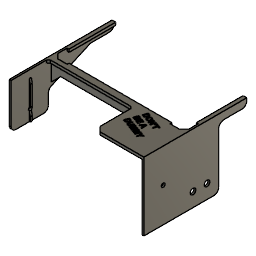
MEANWELL BRACKET (Autodesk Fusion 360 design; units mm, degrees)
Autodesk Fusion 360 part; units mm, degrees
sketch "Sketch1" plane through (0, 0, 0) normal (0, 0, 1) x (1, 0, 0)
  line L0 (95, 0) -> (140, 0)
  line L1 (140, 0) -> (140, 110)
  line L2 (0, 110) -> (0, 0)
  line L3 (90, 5) -> (90, 38)
  line L4 (88, 40) -> (2, 40)
  line L5 (0, 38) -> (0, 0)
  line L6 (0, 110) -> (-2, 110)
  line L7 (-2, 110) -> (-2, 0)
  line L8 (-2, 0) -> (0, 0)
  line L9 (0, 0) -> (0, 110)
  line L10 (140, 0) -> (142, 0)
  line L11 (142, 0) -> (142, 110)
  line L12 (142, 110) -> (140, 110)
  line L13 (140, 110) -> (140, 0)
  line L14 (140, 110) -> (140, 50)
  line L15 (135, 45) -> (5, 45)
  line L16 (0, 50) -> (0, 110)
  line L17 (140, 50) -> (135, 45)
  line L18 (5, 45) -> (0, 50)
  line L19 (90, 38) -> (88, 40)
  line L20 (2, 40) -> (0, 38)
  line L21 (90, 5) -> (95, 0)
  line L22 (0, 45) -> (140, 45)
  line L23 (140, 45) -> (140, 43)
  line L24 (140, 43) -> (0, 43)
  line L25 (0, 43) -> (0, 45)
  line L26 (0, 110) -> (2, 110)
  line L27 (2, 110) -> (2, 60)
  line L28 (2, 60) -> (0, 60)
  line L29 (0, 60) -> (0, 110)
  line L30 (140, 110) -> (138, 110)
  line L31 (138, 110) -> (138, 60)
  line L32 (138, 60) -> (140, 60)
  line L33 (140, 60) -> (140, 110)
  line L34 (5, 45) -> (15, 45)
  line L35 (135, 45) -> (125, 45)
  line L36 (15, 45) -> (125, 45)
  line L37 (125, 45) -> (125, 47)
  line L38 (125, 47) -> (15, 47)
  line L39 (15, 47) -> (15, 45)
  point P0 (90, 0)
  point P1 (90, 40)
  point P2 (0, 40)
  point P3 (140, 45)
  point P4 (0, 45)
  dimension "d1" = 140
  dimension "d2" = 110
  dimension "d3" = 90
  dimension "d4" = 40
  dimension "d5" = 2
  dimension "d6" = 110
  dimension "d7" = 2
  dimension "d8" = 110
  dimension "d9" = 65
  dimension "d10" = 5
  dimension "d11" = 5
  dimension "d12" = 5
  dimension "d13" = 5
  dimension "d14" = 2
  dimension "d15" = 2
  dimension "d16" = 2
  dimension "d17" = 2
  dimension "d18" = 5
  dimension "d19" = 5
  dimension "d22" = 2
  dimension "d23" = 50
  dimension "d24" = 2
  dimension "d25" = 50
  dimension "d26" = 10
  dimension "d27" = 10
  dimension "d28" = 110
  dimension "d29" = 2
  constraint horizontal L0
  constraint vertical L1
  constraint vertical L2
  constraint coincident L2.end L5.end
  constraint vertical L3
  constraint horizontal L4
  constraint vertical L5
  constraint horizontal L6
  constraint vertical L7
  constraint horizontal L8
  constraint vertical L9
  constraint horizontal L10
  constraint vertical L11
  constraint horizontal L12
  constraint vertical L13
  constraint vertical L14
  constraint horizontal L15
  constraint vertical L16
  constraint coincident L1 P3
  constraint coincident P3 L14
  constraint coincident P3 L15
  constraint coincident P4 L15
  constraint coincident P4 L16
  constraint coincident P1 L3
  constraint coincident P1 L4
  constraint coincident P2 L4
  constraint coincident P2 L5
  constraint coincident P0 L3
  constraint coincident L0 P0
  constraint horizontal L22
  constraint vertical L23
  constraint horizontal L24
  constraint vertical L25
  constraint coincident L13 L23.end
  constraint coincident P4 L22.start
  constraint horizontal L26
  constraint vertical L27
  constraint horizontal L28
  constraint vertical L29
  constraint horizontal L30
  constraint vertical L31
  constraint horizontal L32
  constraint vertical L33
  constraint parallel L22 L34
  constraint parallel L22 L35
  constraint horizontal L36
  constraint vertical L37
  constraint horizontal L38
  constraint vertical L39
  measures "d1" distance of L2.end L0.end
  measures "d2" distance of L2.end L2.start
  measures "d3" distance of L2.end P0
  measures "d4" distance of L2.end P2
  measures "d5" distance of L2.start L6.end
  measures "d6" distance of L2.start L2.end
  measures "d7" distance of L0.end L10.end
  measures "d8" distance of L0.end L1.end
  measures "d9" distance of L2.start L22.start
  measures "d10" distance of P3 L14.end
  measures "d11" distance of P3 L15.start
  measures "d12" distance of P4 L15.end
  measures "d13" distance of P4 L16.start
  measures "d14" distance of P1 L3.end
  measures "d15" distance of P1 L4.start
  measures "d16" distance of P2 L4.end
  measures "d17" distance of P2 L5.start
  measures "d18" distance of P0 L3.start
  measures "d19" distance of P0 L0.start
  measures "d22" distance of L2.start L26.end
  measures "d23" distance of L2.start L28.end
  measures "d24" distance of L1.end L30.end
  measures "d25" distance of L1.end L32.end
  measures "d26" distance of L15.end L34.end
  measures "d27" distance of L15.start L35.end
  measures "d28" distance of L34.end L35.end
  measures "d29" distance of L34.end L38.end
extrude "Extrude1" add sketch "Sketch1" along normal blind 3
extrude "Extrude2" add sketch "Sketch1" against normal blind 10 contours L1 L2 L9 L13 L15 L22 L23 L24 L25 L34 L35 L36
extrude "Extrude3" add sketch "Sketch1" against normal blind 45 contours L1 L10 L11 L12 L13 L14 L23 L33 | L2 L5 L6 L7 L8 L9 L16 L25 L29
sketch "Sketch2" plane through (0, 0, 0) normal (1, 0, 0) x (0, 1, 0)
  line L0 (110, -45) -> (40, -45)
  line L1 (40, -45) -> (40, -25)
  line L2 (85, -5) -> (110, -5)
  line L3 (110, -5) -> (110, -45)
  line L4 (40, -25) -> (85, -5)
  point P0 (40, -5)
  dimension "d34" = 70
  dimension "d35" = 40
  dimension "d36" = 20
  dimension "d37" = 45
  constraint horizontal L0
  constraint vertical L1
  constraint horizontal L2
  constraint vertical L3
  constraint coincident P0 L1
  constraint coincident P0 L2
  measures "d34" distance of L0.start L0.end
  measures "d35" distance of L0.start L2.end
  measures "d36" distance of P0 L1.end
  measures "d37" distance of P0 L2.start
extrude "Extrude4" cut sketch "Sketch2" along normal blind 210 and the other way blind 40
sketch "Sketch3" plane through (0, 0, 0) normal (1, 0, 0) x (0, 1, 0)
  line L0 (0, 0) -> (0, -15)
  line L1 (0, -33.26) -> (0, -15)
  circle A0 centre (20.65, -33.26) radius 2
  line L2 (21.65, -34.9921) -> (21.65, -45)
  line L3 (21.65, -45) -> (20.65, -45)
  line L4 (19.65, -34.9921) -> (19.65, -45)
  line L5 (19.65, -45) -> (20.65, -45)
  line L6 (19.65, -45) -> (21.65, -45)
  line L7 (21.65, -5) -> (19.65, -5)
  line L8 (19.65, -5) -> (19.65, -31.5279)
  line L9 (19.65, -34.9921) -> (19.65, -45)
  line L10 (21.65, -45) -> (21.65, -34.9921)
  line L11 (21.65, -31.5279) -> (21.65, -5)
  dimension "d42" = 15
  dimension "d44" = 18.26
  dimension "d45" = 4
  dimension "d54" = 2
  dimension "d55" = 40
  constraint coincident L0.start origin
  constraint vertical L0
  constraint vertical L1
  constraint vertical L2
  constraint horizontal L3
  constraint vertical L4
  constraint horizontal L5
  constraint horizontal L6
  constraint vertical L10
  constraint horizontal L7
  constraint vertical L8
  constraint coincident A0 L8.end
  constraint coincident A0 L4.start
  constraint collinear L8 L9
  constraint coincident A0 L2.start
  constraint coincident A0 L11.start
  constraint collinear L10 L11
  measures "d42" distance of L0.start L0.end
  measures "d44" distance of L0.end L1.start
  measures "d45" diameter of A0
  measures "d54" distance of L4.end L2.end
  measures "d55" distance of L4.end L7.end
extrude "Extrude5" cut sketch "Sketch3" along normal blind 175 and the other way blind 15 contours A0
fillet "Fillet1" radius 5 10 edges at (141, 40, -45) (141, 40, -25) (141, 85, -5) (141, 110, -5) (141, 0, -45) (-1, 0, -45) (-1, 40, -45) (-1, 40, -25) (-1, 85, -5) (-1, 110, -5)
extrude "Extrude6" add sketch "Sketch3" along normal blind 1 contours A0 L7 L8 L11 | A0 L2 L3 L4 L5 L6 L9 L10
chamfer "Chamfer1" distance 5 distance2 1 1 edges at (1, 20.65, -5) measured on face at (1, 20.6002, -13.7552)
chamfer "Chamfer2" distance 4.5 distance2 1 1 edges at (1, 20.65, -35.26) measured on face at (1, 20.6998, -41.7515)
ref_plane "WorkPlane1" through (70, 55, -21) normal (1, 0, 0) x (0, 1, 0)
mirror "Mirror1" about plane through (70, 55, -21) normal (1, 0, 0) of "Extrude6"
chamfer "Chamfer3" distance 1 distance2 5 1 edges at (139, 20.65, -5) measured on face at (139.6667, 20.9833, -5)
chamfer "Chamfer3" distance 1 distance2 5 1 edges at (139, 20.65, -35.26) measured on face at (140.3333, 19.8274, -31.437)
sketch "Sketch4" plane through (142, 0, 0) normal (1, 0, 0) x (0, 1, 0)
  circle A0 centre (20.65, -33.26) radius 2
  arc A1 (0, -40) -> (5, -45) centre (5, -40) ccw
  line L0 (5, -45) -> (35, -45)
  arc A2 (35, -45) -> (40, -40) centre (35, -40) ccw
  line L1 (40, -40) -> (40, -28.2494)
  arc A3 (42.9693, -23.6803) -> (40, -28.2494) centre (45, -28.2494) ccw
  line L2 (42.9693, -23.6803) -> (84.0304, -5.4309)
  arc A4 (86.0611, -5) -> (84.0304, -5.4309) centre (86.0611, -10) ccw
  line L3 (86.0611, -5) -> (105, -5)
  arc A5 (105, -5) -> (110, 0) centre (105, 0) ccw
  line L4 (110, 0) -> (110, 3)
  line L5 (110, 3) -> (0, 3)
  line L6 (0, 3) -> (0, -40)
  line L7 (0, -40) -> (35, -40)
  line L8 (80, -40) -> (80, -70)
  line L9 (80, -70) -> (0, -70)
  line L10 (0, -70) -> (0, -40)
  line L11 (35, -40) -> (35, -5)
  line L12 (35, -5) -> (80, -5)
  line L13 (80, -5) -> (80, -40)
  line L14 (0, -70) -> (67.5, -70)
  line L15 (67.5, -70) -> (67.5, -55)
  line L16 (67.5, -55) -> (0, -55)
  line L17 (0, -55) -> (0, -70)
  line L18 (67.5, -55) -> (52.5, -55)
  circle A6 centre (52.5, -55) radius 3
  circle A7 centre (67.5, -55) radius 3
  dimension "d68" = 80
  dimension "d69" = 30
  dimension "d70" = 45
  dimension "d71" = 35
  dimension "d76" = 67.5
  dimension "d77" = 15
  dimension "d78" = 15
  dimension "d79" = 6
  dimension "d80" = 6
  constraint horizontal L7
  constraint vertical L8
  constraint horizontal L9
  constraint vertical L10
  constraint coincident A1.start L6.end
  constraint vertical L11
  constraint horizontal L12
  constraint vertical L13
  constraint horizontal L14
  constraint vertical L15
  constraint horizontal L16
  constraint vertical L17
  constraint perpendicular L15 L18
  constraint coincident L18.end A6.centre
  constraint coincident L15.end L16.start
  measures "d68" distance of A1.start L8.start
  measures "d69" distance of A1.start L9.end
  measures "d70" distance of L8.start A2.centre
  measures "d71" distance of L8.start L12.end
  measures "d76" distance of L9.end L14.end
  measures "d77" distance of L9.end L16.end
  measures "d78" distance of L15.end L18.end
  measures "d79" diameter of A6
  measures "d80" diameter of A7
extrude "Extrude7" add sketch "Sketch4" against normal blind 2 contours A1 L0 A2 L1 A3 L2 L8 L9 L10 L13 L15 L16 L18 A6 A7 | L9 L10 L14 L15 L16 L17 L18 A6 A7 | L16 L18 A6 | L16 L18 A6 | L15 L16 L18 A7 | L15 L16 L18 A7
fillet "Fillet2" radius 5 2 edges at (141, 80, -70) (141, 80, -7.2222)
extrude "Extrude8" cut sketch "Sketch4" against normal blind 5 contours L16 L18 A6 | L16 L18 A6 | L15 L16 L18 A7 | L15 L16 L18 A7
sketch "Sketch5" plane through (0, 0, 0) normal (0, 0, 1) x (1, 0, 0)
  line L0 (95.8227, 21.6491) -> (130.7793, 8.9259) construction
  line L1 (130.7793, 8.9259) -> (138.5773, 30.3509) construction
  line L2 (138.5773, 30.3509) -> (103.6207, 43.0741) construction
  line L3 (103.6207, 43.0741) -> (95.8227, 21.6491) construction
  dimension "d83" = 5
  text T0 "DON'T\nBE A\nDUMMY" font "Arial" height 5 bold align left top in box 37.2 x 22.8 at (95.8227, 21.6491) x (0.939693, -0.34202) y (0.34202, 0.939693) spacing 1 kerned
extrude "Extrude9" cut sketch "Sketch5" along normal blind 6 and the other way blind -2 text T0
chamfer "Chamfer4" distance 10 distance2 10 2 edges at (140, 44, -10) (0, 44, -10) measured on face at (46.6667, 43.6667, -10) measured on face at (46.6667, 43.6667, -10)
chamfer "Chamfer5" distance 2 distance2 1 1 edges at (70, 43, 0) measured on face at (125, 14.3333, 0)
equation "d11 = d10"
equation "d13 = d12"
equation "d15 = d14"
equation "d17 = d16"
equation "d19 = d18"
